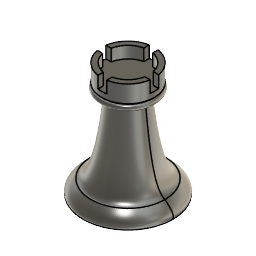
Set sah (Assembly) (Autodesk Fusion 360 archive; units mm, degrees)
design "Tura"
part number: 2026-03-27-15-39-02-789
Autodesk Fusion 360 part; units mm, degrees
sketch "Tura" plane through (0, 0, 0) normal (0, 1, 0) x (1, 0, 0)
  line L0 (0, 0) -> (17, 0)
  line L1 (0, 0) -> (0, -38.5138)
  line L2 (0, -38.5138) -> (0, -35)
  line L3 (0, -38.5138) -> (0, -35)
  line L4 (0, 0) -> (0, -5)
  line L5 (14, -5) -> (0, -5)
  spline S0 degree 5 poles (6.5259, -34) (6.6855, -32.318) (7.0209, -29.0147) (7.5725, -24.2418) (8.412, -18.2671) (9.7194, -11.7648) (11.1016, -7.8229) (12.4226, -5.9311) (13.4497, -5.2188) (14, -5) knots 0 0 0 0 0 0 0.2 0.4 0.6 0.8 1 1 1 1 1 1
  line L6 (12.8092, -5.4735) -> (15.1908, -4.5265)
  spline S1 degree 5 poles (14, -5) (14.3724, -4.7164) (15.065, -4.1591) (15.9469, -3.3525) (16.8041, -2.3367) (17.2264, -1.3701) (17.2496, -0.692) (17.1232, -0.2556) (17.015, -0.0297) (17, 0) knots 0 0 0 0 0 0 0.1 0.2 0.3 0.4 0.415205 0.415205 0.415205 0.415205 0.415205 0.415205
  line L7 (17.1967, -0.3896) -> (16.8033, 0.3896)
  line L8 (0, -37.3622) -> (0, -38.5138)
  line L9 (0, -36) -> (9, -36)
  line L10 (0, -38) -> (0, -36)
  line L11 (8, -40) -> (8, -43)
  line L12 (8, -43) -> (10, -43)
  line L13 (10, -43) -> (10, -36.5)
  line L14 (9.5, -36) -> (9, -36)
  line L15 (0, -36) -> (9.5003, -36)
  line L16 (9.5, -34) -> (0, -34)
  line L17 (0, -34) -> (0, -36)
  arc A0 (9.5005, -34) -> (9.5, -34) centre (9.5, -36.5) ccw
  arc A1 (9.5003, -36) -> (9.5005, -34) centre (9.5003, -35) ccw
  arc A2 (10, -36.5) -> (9.5, -36) centre (9.5, -36.5) ccw
  line L18 (-1.7845, -43) -> (1.4873, -43)
  line L19 (1.4873, -43) -> (1.4873, -38.5138)
  line L20 (1.4873, -38.5138) -> (-1.7845, -38.5138)
  line L21 (-1.7845, -38.5138) -> (-1.7845, -43)
  line L22 (1.4873, -38.5138) -> (8, -38.5138)
  line L23 (8, -38.5138) -> (8, -40)
  point P0 (10, -35)
  dimension "d1" = 17
  dimension "d3" = 10
  dimension "d5" = 3
  dimension "d6" = 2.5
  dimension "d7" = 1
  dimension "d8" = 0.5
  constraint coincident L0.start L1.start
  constraint horizontal L0
  constraint perpendicular L0 L1
  constraint coincident L1 L2.end
  constraint coincident L1 L4.end
  constraint perpendicular L4 L5
  constraint midpoint L5.start L6
  constraint midpoint L0.end L7
  constraint vertical L8
  constraint horizontal L9
  constraint vertical L10
  constraint coincident L1 L9.start
  constraint perpendicular L11 L12
  constraint perpendicular L12 L13
  constraint horizontal L15
  constraint horizontal L16
  constraint vertical L17
  constraint tangent L16 A0
  constraint tangent L15 A1
  constraint tangent A0 A1
  constraint tangent L13 A2
  constraint tangent L14 A2
  constraint coincident S0.start L16
  constraint horizontal L18
  constraint vertical L19
  constraint horizontal L20
  constraint vertical L21
  constraint perpendicular L19 L22
  constraint perpendicular L22 L23
  constraint coincident L20 L1.end
  measures "d1" distance of L0.start L0.end
  measures "d3" distance of L2.end P0
  measures "d5" distance of L11.start L11.end
  measures "d6" radius of A0
  measures "d7" radius of A1
  measures "d8" radius of A2
revolve "Revolve2" add sketch "Tura" angle 360 about axis through (0, 0, 0) along (0, 0, 1) contours L0 L1 L4 L5 S1 | L1 L5 S0 L16 | L1 L2 L3 L9 L15 L16 L17 A0 | L9 L14 L15 A0 A1 | L1 L2 L3 L8 L9 L10 L11 L12 L13 L15 A0 L20 L22 L23 | L9 L13 L14 L15 A0 A2
extrude "Extrude2" cut sketch "Tura" along normal blind 10 contours L18 L19 L20 L21
pattern_circular "C-Pattern1" count 4 over 360 about axis through (0, 0, 0) along (0, 0, 1) of "Extrude2"
named bodies: "Tura"

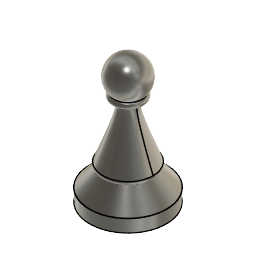
design "Pion"
part number: 2026-03-27-14-13-04-446
Autodesk Fusion 360 part; units mm, degrees
sketch "Pion" plane through (0, 0, 0) normal (0, 1, 0) x (1, 0, 0)
  line L0 (0, 0) -> (12, 0)
  line L1 (12, 0) -> (12, -4) construction
  line L2 (0, 0) -> (0, -40) construction
  line L3 (6, 0) -> (6, -9.5696) construction
  line L4 (0, -30) -> (0, -28) construction
  line L5 (0, -30) -> (4, -30)
  line L6 (0, -28) -> (4, -28)
  arc A0 (4, -30) -> (5, -29) centre (4, -29) ccw
  arc A1 (5, -29) -> (4, -28) centre (4, -29) ccw
  line L7 (12, -4) -> (12, 0)
  line L8 (0, -40) -> (0, 0)
  line L9 (12, -4) -> (0, -4) construction
  line L10 (0, -9.6135) -> (6.9254, -9.6135)
  spline S0 degree 5 poles (7.8558, -10.9801) (7.5549, -11.7439) (6.8618, -13.5183) (5.8277, -16.2235) (4.5513, -19.7052) (3.268, -23.5962) (2.6775, -26.112) (2.6509, -27.3491) (2.8478, -27.8389) (3, -28) knots 0.052342 0.052342 0.052342 0.052342 0.052342 0.052342 0.2 0.4 0.6 0.8 1 1 1 1 1 1
  line L11 (2.6823, -27.6637) -> (3.3177, -28.3363)
  arc A2 (7.8558, -10.9801) -> (6.9254, -9.6135) centre (6.9254, -10.6135) ccw
  spline S1 degree 5 poles (6.9254, -9.6135) (7.1769, -9.3353) (7.6663, -8.794) (8.3596, -8.027) (9.2012, -7.0961) (10.1055, -6.0957) (10.8484, -5.274) (11.4156, -4.6465) (11.7977, -4.2238) (11.9996, -4.0005) (12.0478, -3.9472) (12.0208, -3.977) (12.0038, -3.9958) (12, -4) (12, -4) knots 0 0 0 0 0 0 0.1 0.2 0.3 0.4 0.5 0.6 0.7 0.8 0.9 1 1 1 1 1 1
  line L12 (12.2553, -4.7429) -> (11.7447, -3.257)
  arc A3 (0, -39.9814) -> (4.3789, -29.9254) centre (0, -34) ccw
  dimension "d1" = 12
  dimension "d2" = 4
  dimension "d3" = 40
  dimension "d5" = 2
  dimension "d6" = 1
  dimension "d7" = 1
  constraint coincident L0.start L2.start
  constraint horizontal L0
  constraint perpendicular L0 L1
  constraint perpendicular L0 L2
  constraint midpoint L0 L3.start
  constraint perpendicular L0 L3
  constraint coincident L2 L4.start
  constraint parallel L2 L4
  constraint perpendicular L4 L5
  constraint perpendicular L4 L6
  constraint tangent L5 A0
  constraint tangent L6 A1
  constraint equal A0 A1
  constraint coincident A0.end A1.start
  constraint coincident L1 L7.start
  constraint coincident L2 L9.end
  constraint perpendicular L2 L9
  constraint coincident L8 L10.start
  constraint perpendicular L3 L10
  constraint coincident L6 S0.end
  constraint midpoint S0.end L11
  constraint tangent L10 A2
  constraint tangent S0 A2
  constraint midpoint L1.end L12
  constraint coincident L2 A3.centre
  constraint coincident L2 A3.start
  constraint coincident A0 A3.end
  measures "d1" distance of L0.start L0.end
  measures "d2" distance of L0.end L1.end
  measures "d3" distance of L0.start L2.end
  measures "d5" distance of L4.start L4.end
  measures "d6" radius of A0
  measures "d7" radius of A2
revolve "Revolve1" add sketch "Pion" angle 360 about axis through (0, 0, 40) along (0, 0, -1)
named bodies: "Pion"

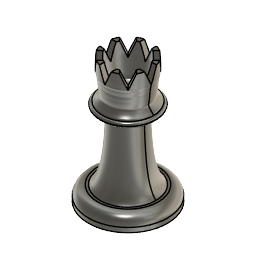
design "Regina"
part number: 2026-03-27-17-57-06-025
Autodesk Fusion 360 part; units mm, degrees
sketch "Regina" plane through (0, 0, 0) normal (0, 1, 0) x (1, 0, 0)
  line L0 (0, 0) -> (17, 0)
  line L1 (0, 0) -> (0, -41)
  line L2 (17, 0) -> (17, -2)
  line L3 (13, -6) -> (0, -6)
  line L4 (0, -41) -> (0, -39.2065) construction
  line L5 (3.0623, -35) -> (0, -35)
  line L6 (0, -35) -> (0, -39.2065)
  arc A0 (13, -6) -> (17, -2) centre (13, -2) ccw
  line L7 (0, -39) -> (0, -41)
  arc A1 (10.0008, -39) -> (10, -39) centre (10, -40) ccw
  line L8 (3.0623, -35) -> (10.9377, -35)
  line L9 (0, -37.1033) -> (10.9434, -37.1033)
  line L10 (11.9419, -36.0482) -> (11.9362, -35.945)
  arc A2 (10.9434, -37.1033) -> (11.9419, -36.0482) centre (10.9434, -36.1033) ccw
  arc A3 (11.9362, -35.945) -> (10.9377, -35) centre (10.9377, -36) ccw
  spline S0 degree 5 poles (0, -41) (0.2083, -40.9398) (0.6157, -40.8267) (1.1995, -40.6787) (1.9231, -40.5249) (2.7363, -40.4049) (3.4584, -40.3568) (4.0905, -40.3792) (4.6342, -40.4699) (5.0924, -40.6251) (5.4693, -40.8395) (5.7707, -41.1057) (6.0047, -41.4142) (6.1808, -41.7532) (6.3098, -42.1104) (6.403, -42.4744) (6.4712, -42.8361) (6.5241, -43.1902) (6.5701, -43.5357) (6.6153, -43.8747) (6.6643, -44.2102) (6.7194, -44.545) (6.7805, -44.8795) (6.8453, -45.2114) (6.9105, -45.5373) (6.9731, -45.8546) (7.0311, -46.1635) (7.085, -46.4688) (7.138, -46.7792) (7.1936, -47.1039) (7.2549, -47.4491) (7.3229, -47.8152) (7.3951, -48.1929) (7.4664, -48.5665) (7.531, -48.9193) (7.5841, -49.2385) (7.6231, -49.5189) (7.6499, -49.7696) (7.6697, -50.0089) (7.6883, -50.2559) (7.711, -50.5249) (7.7399, -50.8159) (7.7746, -51.1193) (7.8131, -51.4217) (7.8528, -51.7111) (7.8909, -51.9831) (7.9257, -52.2421) (7.9554, -52.4973) (7.9791, -52.7592) (7.9959, -53.0363) (8.0054, -53.3331) (8.007, -53.5884) (8.0048, -53.7902) (8.0019, -53.9293) (8, -54) knots 0 0 0 0 0 0 0.02 0.04 0.06 0.08 0.1 0.12 0.14 0.16 0.18 0.2 0.22 0.24 0.26 0.28 0.3 0.32 0.34 0.36 0.38 0.4 0.42 0.44 0.46 0.48 0.5 0.52 0.54 0.56 0.58 0.6 0.62 0.64 0.66 0.68 0.7 0.72 0.74 0.76 0.78 0.8 0.82 0.84 0.86 0.88 0.9 0.92 0.94 0.96 0.98 1 1 1 1 1 1
  line L11 (8, -54) -> (10, -54)
  spline S1 degree 5 poles (10, -54) (10.0003, -53.9643) (10.0009, -53.893) (10.0015, -53.7863) (10.0021, -53.6443) (10.0022, -53.4675) (10.0017, -53.2913) (10.0008, -53.1155) (9.9996, -52.94) (9.9984, -52.7646) (9.9975, -52.5889) (9.9973, -52.4126) (9.9978, -52.2353) (9.9993, -52.057) (10.0013, -51.8776) (10.0035, -51.6974) (10.0048, -51.5172) (10.0047, -51.3382) (10.003, -51.1625) (9.9998, -50.9932) (9.9971, -50.8349) (9.9962, -50.6912) (9.997, -50.5614) (9.999, -50.4427) (10.001, -50.3302) (10.0023, -50.218) (10.0027, -50.0997) (10.0018, -49.9699) (9.9999, -49.825) (9.9968, -49.6648) (9.9924, -49.4929) (9.9865, -49.3152) (9.9792, -49.1386) (9.971, -48.9695) (9.9624, -48.8122) (9.9548, -48.6674) (9.9498, -48.5327) (9.9485, -48.4043) (9.9508, -48.2781) (9.9552, -48.1515) (9.9578, -48.0242) (9.9542, -47.8975) (9.9404, -47.7728) (9.9147, -47.6506) (9.8786, -47.5297) (9.8367, -47.407) (9.7944, -47.2791) (9.7566, -47.1427) (9.7263, -46.9962) (9.7031, -46.8396) (9.685, -46.6745) (9.6688, -46.5033) (9.6514, -46.3293) (9.6302, -46.1561) (9.6043, -45.9872) (9.5742, -45.8253) (9.5412, -45.6726) (9.5073, -45.5295) (9.4745, -45.3949) (9.4447, -45.2651) (9.4194, -45.1349) (9.3997, -44.999) (9.3857, -44.8526) (9.3769, -44.6934) (9.3716, -44.522) (9.3676, -44.341) (9.3626, -44.1544) (9.3546, -43.9664) (9.3422, -43.781) (9.3251, -43.6008) (9.3045, -43.4266) (9.2819, -43.2581) (9.2593, -43.0941) (9.2383, -42.9328) (9.22, -42.7721) (9.2045, -42.6102) (9.1909, -42.4455) (9.1778, -42.2768) (9.1638, -42.1036) (9.1473, -41.9261) (9.1273, -41.7453) (9.1032, -41.5633) (9.0751, -41.3824) (9.0431, -41.2052) (9.0082, -41.0339) (8.9713, -40.8699) (8.934, -40.7138) (8.898, -40.5652) (8.8656, -40.4228) (8.8396, -40.2852) (8.8232, -40.1502) (8.8205, -40.016) (8.8353, -39.881) (8.8703, -39.7444) (8.9259, -39.607) (8.9989, -39.4716) (9.0821, -39.3435) (9.1671, -39.2279) (9.2462, -39.1285) (9.3149, -39.0458) (9.3748, -38.9745) (9.4331, -38.9045) (9.4986, -38.825) (9.5792, -38.7278) (9.6773, -38.6117) (9.7913, -38.4807) (9.9167, -38.342) (10.0475, -38.2039) (10.1775, -38.0737) (10.302, -37.9554) (10.4179, -37.8484) (10.5238, -37.7498) (10.6193, -37.655) (10.7045, -37.5589) (10.7796, -37.4576) (10.8449, -37.3489) (10.8892, -37.2551) (10.918, -37.1808) (10.9352, -37.1294) (10.9434, -37.1033) knots 0 0 0 0 0 0 0.00869565 0.0173913 0.02608696 0.03478261 0.04347826 0.05217391 0.06086957 0.06956522 0.07826087 0.08695652 0.09565217 0.10434783 0.11304348 0.12173913 0.13043478 0.13913043 0.14782609 0.15652174 0.16521739 0.17391304 0.1826087 0.19130435 0.2 0.20869565 0.2173913 0.22608696 0.23478261 0.24347826 0.25217391 0.26086957 0.26956522 0.27826087 0.28695652 0.29565217 0.30434783 0.31304348 0.32173913 0.33043478 0.33913043 0.34782609 0.35652174 0.36521739 0.37391304 0.3826087 0.39130435 0.4 0.40869565 0.4173913 0.42608696 0.43478261 0.44347826 0.45217391 0.46086957 0.46956522 0.47826087 0.48695652 0.49565217 0.50434783 0.51304348 0.52173913 0.53043478 0.53913043 0.54782609 0.55652174 0.56521739 0.57391304 0.5826087 0.59130435 0.6 0.60869565 0.6173913 0.62608696 0.63478261 0.64347826 0.65217391 0.66086957 0.66956522 0.67826087 0.68695652 0.69565217 0.70434783 0.71304348 0.72173913 0.73043478 0.73913043 0.74782609 0.75652174 0.76521739 0.77391304 0.7826087 0.79130435 0.8 0.80869565 0.8173913 0.82608696 0.83478261 0.84347826 0.85217391 0.86086957 0.86956522 0.87826087 0.88695652 0.89565217 0.90434783 0.91304348 0.92173913 0.93043478 0.93913043 0.94782609 0.95652174 0.96521739 0.97391304 0.9826087 0.99130435 1 1 1 1 1 1
  line L12 (10.0315, -52.8303) -> (9.9685, -49.1697)
  line L13 (-1.0096, -55) -> (-3, -55) construction
  line L14 (-3, -55) -> (-1.0096, -55) construction
  line L15 (-3, -55) -> (3, -55)
  line L16 (-3, -55) -> (0, -48)
  line L17 (0, -48) -> (3, -55)
  spline S2 degree 5 poles (7, -35) (7.0241, -33.463) (7.0927, -30.4328) (7.257, -26.0189) (7.6072, -20.4148) (8.3706, -14.1076) (9.4058, -9.9718) (10.541, -7.6389) (11.4828, -6.4802) (12, -6) knots 0 0 0 0 0 0 0.2 0.4 0.6 0.8 1 1 1 1 1 1
  line L18 (10.7838, -7.1292) -> (13.2162, -4.8708)
  point P0 (5.6353, -41)
  point P1 (6.4544, -42.7608)
  point P2 (6.7049, -44.4511)
  point P3 (7, -46)
  point P4 (7.2683, -47.5188)
  point P5 (7.5908, -49.2968)
  point P6 (7.6929, -50.3049)
  point P7 (7.8324, -51.5607)
  point P8 (7.9675, -52.6412)
  point P9 (10, -53)
  point P10 (10, -52)
  point P11 (10, -51)
  point P12 (10, -50.3822)
  point P13 (10, -49.8453)
  point P14 (9.9685, -48.9259)
  point P15 (9.951, -48.2884)
  point P16 (9.9322, -47.743)
  point P17 (9.7687, -47.1812)
  point P18 (9.6508, -46.3325)
  point P19 (9.5, -45.5)
  point P20 (9.3886, -44.8701)
  point P21 (9.3475, -43.8691)
  point P22 (9.2378, -42.9231)
  point P23 (9.1555, -42.0181)
  point P24 (9, -41)
  point P25 (8.8377, -40.2561)
  point P26 (8.9191, -39.6317)
  point P27 (9.2788, -39.0895)
  point P28 (9.5164, -38.8037)
  point P29 (10.1272, -38.125)
  point P30 (10.6702, -37.5956)
  dimension "d1" = 17
  dimension "d4" = 4
  dimension "d7" = 1
  constraint coincident L0.start L1.start
  constraint horizontal L0
  constraint perpendicular L0 L1
  constraint perpendicular L0 L2
  constraint coincident L1 L3.end
  constraint perpendicular L1 L3
  constraint coincident L1 L4.end
  constraint horizontal L5
  constraint vertical L6
  constraint tangent L2 A0
  constraint tangent L3 A0
  constraint vertical L7
  constraint parallel L5 L8
  constraint midpoint L6 L9.start
  constraint perpendicular L1 L9
  constraint tangent L9 A2
  constraint tangent L10 A2
  constraint tangent L8 A3
  constraint tangent L10 A3
  constraint equal A2 A3
  constraint horizontal L11
  constraint midpoint P11 L12
  constraint horizontal L13
  constraint parallel L14 L15
  constraint midpoint L8 S2.start
  constraint coincident L3 S2.end
  constraint midpoint S2.end L18
  measures "d1" distance of L0.start L0.end
  measures "d4" radius of A0
  measures "d7" radius of A2
revolve "Revolve2" add sketch "Regina" angle 360 about axis through (0, 0, 0) along (0, 0, 1) contours L0 L1 L2 L3 A0 | L1 L3 L5 L8 S2 | L1 L5 L6 L8 L9 L10 A2 A3 | L1 L6 L7 L9 S0 L11 S1
extrude "Extrude3" cut sketch "Regina" along normal blind 14 contours L15 L16 L17
pattern_circular "C-Pattern3" count 8 over 360 about axis through (0, 0, 37.1033) along (0, 0, 1) of "Extrude3"
named bodies: "Regina"

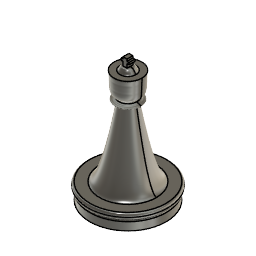
design "Rege"
part number: 2026-03-27-19-00-09-599
Autodesk Fusion 360 part; units mm, degrees
sketch "Rege" plane through (0, 0, 0) normal (0, 1, 0) x (1, 0, 0)
  line L0 (0, 0) -> (19, 0)
  line L1 (0, 0) -> (0, -60)
  line L2 (0, 0) -> (19, 0)
  line L3 (19, 0) -> (19, -4)
  line L4 (18, -5) -> (0, -5)
  line L5 (0, -5) -> (0, 0)
  line L6 (0, -5) -> (19, -5)
  line L7 (18.9974, -7.9995) -> (0, -7.9995)
  line L8 (0, -7.9995) -> (0, -5)
  arc A0 (18.9974, -7.9995) -> (19.8649, -6.502) centre (18.9974, -6.9995) ccw
  arc A1 (19.8649, -6.502) -> (19, -5) centre (19, -6) ccw
  arc A2 (18, -5) -> (19, -4) centre (18, -4) ccw
  line L9 (0, -60) -> (0, -48)
  line L10 (0, -60) -> (0, -40)
  line L11 (0, -37.8406) -> (0, -40)
  line L12 (0, -40) -> (0, -43.0218)
  line L13 (0, -44.611) -> (4.5124, -44.611)
  line L14 (0, -43.0218) -> (0, -44.611)
  spline S0 degree 5 poles (4.3, -42.4) (4.5854, -40.7333) (5.1533, -37.4872) (5.9962, -32.8797) (7.1016, -27.2682) (8.4509, -21.2027) (9.7649, -16.1777) (11.041, -12.29) (12.2781, -9.611) (13.4785, -8.1257) (14.6503, -7.6865) (15.5797, -7.8283) (16.2833, -7.9459) (16.757, -7.9878) (16.995, -7.9995) knots 0 0 0 0 0 0 0.1 0.2 0.3 0.4 0.5 0.6 0.7 0.8 0.9 1 1 1 1 1 1
  line L15 (13.1828, -7.8119) -> (20.8072, -8.1871)
  line L16 (0, -62) -> (1, -62)
  line L17 (1, -62) -> (1, -61)
  line L18 (1, -61) -> (2, -61)
  line L19 (2, -61) -> (2, -60)
  line L20 (2, -60) -> (1, -60)
  line L21 (1, -60) -> (1, -58)
  line L22 (1, -58) -> (0, -58)
  line L23 (0, -60) -> (0, -62)
  spline S1 degree 5 poles (1, -58) (1.0261, -58.002) (1.0784, -58.0057) (1.157, -58.0102) (1.2626, -58.0139) (1.3953, -58.0148) (1.5285, -58.0119) (1.6613, -58.0054) (1.7923, -57.9951) (1.9194, -57.9812) (2.0399, -57.9637) (2.1511, -57.9425) (2.2509, -57.9175) (2.3386, -57.8882) (2.4148, -57.8537) (2.4825, -57.8127) (2.5449, -57.7643) (2.6056, -57.7078) (2.6673, -57.6437) (2.731, -57.5736) (2.7967, -57.4997) (2.8633, -57.4243) (2.9296, -57.3492) (2.9944, -57.2749) (3.0568, -57.2001) (3.1167, -57.1232) (3.174, -57.0419) (3.2294, -56.9548) (3.284, -56.8615) (3.3394, -56.7629) (3.3975, -56.6609) (3.4601, -56.5577) (3.529, -56.4553) (3.6054, -56.3556) (3.6901, -56.2596) (3.7837, -56.1679) (3.8657, -56.0984) (3.9313, -56.0483) (3.9768, -56.016) (4, -56) knots 0 0 0 0 0 0 0.028571 0.057143 0.085714 0.114286 0.142857 0.171429 0.2 0.228571 0.257143 0.285714 0.314286 0.342857 0.371429 0.4 0.428571 0.457143 0.485714 0.514286 0.542857 0.571429 0.6 0.628571 0.657143 0.685714 0.714286 0.742857 0.771429 0.8 0.828571 0.857143 0.885714 0.914286 0.942857 0.971429 1 1 1 1 1 1
  line L24 (4, -56) -> (7, -56)
  spline S2 degree 5 poles (4.5124, -44.611) (4.5363, -44.6464) (4.5836, -44.7159) (4.6528, -44.8164) (4.7418, -44.9431) (4.8473, -45.0892) (4.9477, -45.2239) (5.0436, -45.3482) (5.1363, -45.4642) (5.2275, -45.575) (5.3196, -45.6843) (5.4142, -45.7953) (5.5127, -45.9104) (5.6149, -46.0299) (5.7192, -46.1519) (5.823, -46.2737) (5.9236, -46.3925) (6.0183, -46.5068) (6.1055, -46.6173) (6.1842, -46.7269) (6.2544, -46.8393) (6.3163, -46.9576) (6.3707, -47.0832) (6.4186, -47.2156) (6.461, -47.3527) (6.499, -47.4924) (6.5334, -47.6329) (6.5651, -47.7744) (6.5944, -47.9176) (6.6216, -48.0643) (6.6465, -48.216) (6.6688, -48.3742) (6.6877, -48.5393) (6.7026, -48.7114) (6.7132, -48.8904) (6.7193, -49.0755) (6.722, -49.266) (6.7227, -49.4608) (6.7233, -49.6587) (6.7255, -49.8585) (6.7307, -50.0587) (6.7396, -50.2577) (6.7516, -50.4538) (6.7655, -50.6453) (6.7796, -50.831) (6.7923, -51.0103) (6.8026, -51.1836) (6.8102, -51.3526) (6.8158, -51.5199) (6.8207, -51.6886) (6.8259, -51.8614) (6.8323, -52.0401) (6.8399, -52.2248) (6.8478, -52.4137) (6.8548, -52.6045) (6.8598, -52.7945) (6.8622, -52.9814) (6.8623, -53.1645) (6.8615, -53.3447) (6.862, -53.5237) (6.866, -53.704) (6.8752, -53.8879) (6.8906, -54.0768) (6.9114, -54.2708) (6.9362, -54.469) (6.9623, -54.6696) (6.9871, -54.8706) (7.008, -55.0699) (7.0229, -55.266) (7.0304, -55.4576) (7.0296, -55.6442) (7.0222, -55.7893) (7.0126, -55.8956) (7.0045, -55.9654) (7, -56) knots 0 0 0 0 0 0 0.01428571 0.02857143 0.04285714 0.05714286 0.07142857 0.08571429 0.1 0.11428571 0.12857143 0.14285714 0.15714286 0.17142857 0.18571429 0.2 0.21428571 0.22857143 0.24285714 0.25714286 0.27142857 0.28571429 0.3 0.31428571 0.32857143 0.34285714 0.35714286 0.37142857 0.38571429 0.4 0.41428571 0.42857143 0.44285714 0.45714286 0.47142857 0.48571429 0.5 0.51428571 0.52857143 0.54285714 0.55714286 0.57142857 0.58571429 0.6 0.61428571 0.62857143 0.64285714 0.65714286 0.67142857 0.68571429 0.7 0.71428571 0.72857143 0.74285714 0.75714286 0.77142857 0.78571429 0.8 0.81428571 0.82857143 0.84285714 0.85714286 0.87142857 0.88571429 0.9 0.91428571 0.92857143 0.94285714 0.95714286 0.97142857 0.98571429 1 1 1 1 1 1
  line L25 (11, -41.5218) -> (11, -41.5)
  line L26 (0, -42.4) -> (4.7, -42.4)
  line L27 (0, -44.611) -> (4.5124, -44.611)
  spline S3 degree 5 poles (4.5124, -44.611) (4.5154, -44.5998) (4.5227, -44.5779) (4.5373, -44.5462) (4.5641, -44.5064) (4.6099, -44.4604) (4.6672, -44.4181) (4.7346, -44.3788) (4.8099, -44.3414) (4.8897, -44.3046) (4.971, -44.2668) (5.0508, -44.2273) (5.1275, -44.1854) (5.2013, -44.1421) (5.274, -44.0992) (5.3486, -44.0588) (5.428, -44.0231) (5.514, -43.9937) (5.6068, -43.9707) (5.7039, -43.9528) (5.8016, -43.9376) (5.8956, -43.9226) (5.9825, -43.9055) (6.0599, -43.8852) (6.1285, -43.8623) (6.1907, -43.8388) (6.2497, -43.8166) (6.3077, -43.7971) (6.3652, -43.7795) (6.4194, -43.7609) (6.4664, -43.7371) (6.502, -43.7046) (6.5232, -43.6622) (6.5297, -43.6119) (6.523, -43.5581) (6.5052, -43.5053) (6.4782, -43.4569) (6.4424, -43.4129) (6.397, -43.3711) (6.3413, -43.3284) (6.2746, -43.2819) (6.1975, -43.2306) (6.1117, -43.1754) (6.0196, -43.1187) (5.924, -43.0634) (5.8277, -43.0123) (5.7327, -42.9673) (5.64, -42.9285) (5.5496, -42.8945) (5.4611, -42.8628) (5.3731, -42.8306) (5.2847, -42.7948) (5.1946, -42.7526) (5.1021, -42.7024) (5.0067, -42.6428) (4.9081, -42.5731) (4.8266, -42.5091) (4.7639, -42.4564) (4.7214, -42.4191) (4.7, -42.4) knots 0 0 0 0 0 0 0.018182 0.036364 0.054545 0.072727 0.090909 0.109091 0.127273 0.145455 0.163636 0.181818 0.2 0.218182 0.236364 0.254545 0.272727 0.290909 0.309091 0.327273 0.345455 0.363636 0.381818 0.4 0.418182 0.436364 0.454545 0.472727 0.490909 0.509091 0.527273 0.545455 0.563636 0.581818 0.6 0.618182 0.636364 0.654545 0.672727 0.690909 0.709091 0.727273 0.745455 0.763636 0.781818 0.8 0.818182 0.836364 0.854545 0.872727 0.890909 0.909091 0.927273 0.945455 0.963636 0.981818 1 1 1 1 1 1
  line L28 (0, -62) -> (-1, -62)
  line L29 (-1, -62) -> (-1, -61)
  line L30 (-1, -61) -> (-2, -61)
  line L31 (-2, -61) -> (-2, -60)
  line L32 (-2, -60) -> (-1, -60)
  line L33 (-1, -60) -> (-1, -58)
  line L34 (-1, -58) -> (0, -58)
  point P0 (14.0855, -7.9995)
  point P1 (1.7236, -58)
  point P2 (2.3, -57.9)
  point P3 (2.6058, -57.706)
  point P4 (2.91, -57.3713)
  point P5 (3.2, -57)
  point P6 (3.5, -56.5)
  point P7 (5.0617, -45.3702)
  point P8 (5.4826, -45.8753)
  point P9 (5.9597, -46.4365)
  point P10 (6.2959, -46.9218)
  point P11 (6.5, -47.5)
  point P12 (6.6352, -48.1496)
  point P13 (6.716, -48.9897)
  point P14 (6.7321, -50.0721)
  point P15 (6.7967, -51.0899)
  point P16 (6.8291, -51.9461)
  point P17 (6.8614, -52.9478)
  point P18 (6.8775, -53.9009)
  point P19 (7, -55)
  point P20 (4.7, -44.4)
  point P21 (5.1, -44.2)
  point P22 (5.5, -44)
  point P23 (6, -43.9)
  point P24 (6.3, -43.8)
  point P25 (6.5, -43.7)
  point P26 (6.5, -43.5)
  point P27 (6.3, -43.3)
  point P28 (5.8, -43)
  point P29 (5.3, -42.8)
  dimension "d1" = 19
  dimension "d2" = 1
  dimension "d3" = 20
  dimension "d5" = 2
  constraint coincident L0.start L1.start
  constraint horizontal L0
  constraint perpendicular L0 L1
  constraint horizontal L2
  constraint vertical L3
  constraint horizontal L4
  constraint vertical L5
  constraint horizontal L6
  constraint horizontal L7
  constraint vertical L8
  constraint tangent L7 A0
  constraint tangent L6 A1
  constraint equal A0 A1
  constraint coincident A0.end A1.start
  constraint tangent L3 A2
  constraint tangent L4 A2
  constraint equal A0 A2
  constraint coincident L1 L9.end
  constraint parallel L1 L10
  constraint vertical L11
  constraint vertical L12
  constraint coincident L1 L12.end
  constraint horizontal L13
  constraint vertical L14
  constraint coincident L1 L13.start
  constraint coincident L7 S0.end
  constraint midpoint S0.end L15
  constraint perpendicular L10 L16
  constraint perpendicular L16 L17
  constraint perpendicular L17 L18
  constraint perpendicular L18 L19
  constraint perpendicular L17 L20
  constraint perpendicular L20 L21
  constraint coincident L10 L22.end
  constraint perpendicular L16 L23
  constraint perpendicular L9 L24
  constraint coincident L7 P0
  constraint coincident L1 L26.start
  constraint perpendicular L12 L26
  constraint perpendicular L1 L27
  constraint coincident S0.start L26
  constraint perpendicular L23 L28
  constraint perpendicular L28 L29
  constraint perpendicular L29 L30
  constraint perpendicular L30 L31
  constraint perpendicular L31 L32
  constraint perpendicular L32 L33
  constraint perpendicular L10 L34
  measures "d1" distance of L0.start L0.end
  measures "d2" radius of A0
  measures "d3" distance of L1.end L10.end
  measures "d5" distance of L20.end L21.end
revolve "Revolve1" add sketch "Rege" angle 360 about axis through (0, 0, 0) along (0, 0, 1) contours L0 L1 L2 L3 L4 L5 L6 A2 | L1 L4 L6 L7 L8 A0 A1 S0 L15 | L1 L7 L10 L11 L12 S0 L26 | L1 L10 L12 L13 L14 L26 L27 S3 | L1 L9 L10 L13 L22 S1 L24 S2 L27 picked at (12.3333, -1.6667) picked at (10.6952, -5.9998) picked at (2.9652, -21.8232) picked at (2.9417, -43.3323) picked at (3.5718, -50.9916)
extrude "Extrude1" add sketch "Rege" along normal blind 1.5 and the other way blind 1.5 contours L1 L9 L10 L16 L17 L18 L19 L20 L21 L22 L23 | L1 L9 L10 L23 L28 L29 L30 L31 L32 L33 L34 picked at (0.3333, -61) picked at (-0.3333, -61)
named bodies: "Rege"

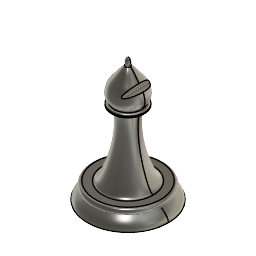
design "Nebun"
part number: 2026-03-27-16-39-54-698
Autodesk Fusion 360 part; units mm, degrees
sketch "Nebun" plane through (0, 0, 0) normal (0, 1, 0) x (1, 0, 0)
  line L0 (0, 0) -> (0, -46.4544)
  line L1 (0, -46.4544) -> (0, -45.1268) construction
  line L2 (0, -35) -> (0, -45.1268)
  arc A0 (0, -46.4544) -> (1, -46) centre (0, -45.1268) ccw
  line L3 (0, -32.0025) -> (3.4069, -32.0025)
  line L4 (3.4069, -32.0025) -> (5.4675, -32.0025)
  line L5 (9.9478, -6.4764) -> (0, -6.4764)
  line L6 (0, -49) -> (0, -46.4544)
  spline S0 degree 5 poles (0, -46.4544) (0.0754, -46.4311) (0.2198, -46.3948) (0.4172, -46.3713) (0.641, -46.4028) (0.8509, -46.5512) (0.9847, -46.8088) (1.036, -47.1672) (1.0017, -47.5979) (0.8824, -48.0528) (0.6792, -48.4775) (0.4497, -48.7506) (0.2397, -48.8993) (0.0827, -48.971) (0, -49) knots 0 0 0 0 0 0 0.1 0.2 0.3 0.4 0.5 0.6 0.7 0.8 0.9 1 1 1 1 1 1
  line L7 (0.2729, -48.9043) -> (-0.2729, -49.0957)
  line L8 (0, 0) -> (16, 0)
  line L9 (0, -6.4764) -> (12.9366, -6.4764)
  line L10 (12.9366, -4.0764) -> (0, -4.0764)
  line L11 (0, -4.0764) -> (0, -6.4764)
  arc A1 (12.9366, -6.4764) -> (14.1366, -5.2855) centre (12.9366, -5.2764) ccw
  arc A2 (14.1366, -5.2855) -> (12.9366, -4.0764) centre (12.9366, -5.2764) ccw
  spline S1 degree 5 poles (12.9366, -4.0764) (13.1271, -3.9343) (13.5002, -3.6476) (14.0361, -3.2102) (14.7, -2.6114) (15.4041, -1.8243) (15.8034, -1.1441) (15.9642, -0.5913) (16, -0.2008) (16, 0) knots 0 0 0 0 0 0 0.2 0.4 0.6 0.8 1 1 1 1 1 1
  line L12 (16, -0.463) -> (16, 0.463)
  line L13 (0, -33.5564) -> (5.4675, -33.5564)
  spline S2 degree 5 poles (1, -46) (1.0428, -45.9606) (1.127, -45.8825) (1.2496, -45.7674) (1.4055, -45.6178) (1.5877, -45.4373) (1.7578, -45.2628) (1.917, -45.0931) (2.0669, -44.9266) (2.2103, -44.7605) (2.3506, -44.5914) (2.4916, -44.4159) (2.6365, -44.2312) (2.7873, -44.0357) (2.9446, -43.8302) (3.107, -43.6175) (3.2717, -43.4017) (3.4359, -43.1875) (3.5967, -42.9791) (3.7521, -42.7796) (3.9018, -42.5897) (4.047, -42.4082) (4.1899, -42.2323) (4.3327, -42.0587) (4.4778, -41.884) (4.6264, -41.705) (4.7787, -41.5199) (4.9342, -41.3276) (5.0913, -41.128) (5.2481, -40.9217) (5.402, -40.7106) (5.5503, -40.4973) (5.6899, -40.285) (5.8185, -40.0766) (5.9341, -39.8743) (6.0357, -39.6789) (6.1236, -39.4894) (6.1993, -39.3029) (6.2652, -39.1158) (6.3237, -38.9245) (6.3773, -38.726) (6.4282, -38.519) (6.4776, -38.3035) (6.5263, -38.081) (6.5739, -37.8538) (6.619, -37.6253) (6.6591, -37.3992) (6.691, -37.1796) (6.712, -36.9697) (6.7203, -36.7711) (6.7158, -36.5835) (6.701, -36.4038) (6.6795, -36.2273) (6.6541, -36.05) (6.6259, -35.8693) (6.5924, -35.686) (6.5483, -35.5037) (6.4876, -35.3265) (6.4054, -35.1579) (6.3, -34.9985) (6.1733, -34.8459) (6.0294, -34.6971) (5.8729, -34.5499) (5.7084, -34.4052) (5.5382, -34.2692) (5.363, -34.1508) (5.1825, -34.0577) (4.9957, -33.9928) (4.8019, -33.95) (4.6011, -33.911) (4.3938, -33.8513) (4.2232, -33.7669) (4.0929, -33.6741) (4.0051, -33.598) (3.9609, -33.5564) knots 0 0 0 0 0 0 0.01428571 0.02857143 0.04285714 0.05714286 0.07142857 0.08571429 0.1 0.11428571 0.12857143 0.14285714 0.15714286 0.17142857 0.18571429 0.2 0.21428571 0.22857143 0.24285714 0.25714286 0.27142857 0.28571429 0.3 0.31428571 0.32857143 0.34285714 0.35714286 0.37142857 0.38571429 0.4 0.41428571 0.42857143 0.44285714 0.45714286 0.47142857 0.48571429 0.5 0.51428571 0.52857143 0.54285714 0.55714286 0.57142857 0.58571429 0.6 0.61428571 0.62857143 0.64285714 0.65714286 0.67142857 0.68571429 0.7 0.71428571 0.72857143 0.74285714 0.75714286 0.77142857 0.78571429 0.8 0.81428571 0.82857143 0.84285714 0.85714286 0.87142857 0.88571429 0.9 0.91428571 0.92857143 0.94285714 0.95714286 0.97142857 0.98571429 1 1 1 1 1 1
  line L14 (5.5565, -35.059) -> (2.3653, -32.0538)
  line L15 (6.4675, -32.5564) -> (6.4675, -33.0025)
  arc A3 (5.4675, -33.5564) -> (6.4675, -32.5564) centre (5.4675, -32.5564) ccw
  arc A4 (6.4675, -33.0025) -> (5.4675, -32.0025) centre (5.4675, -33.0025) ccw
  spline S3 degree 5 poles (4.4372, -32.0025) (4.3926, -31.7636) (4.3089, -31.2754) (4.1994, -30.5122) (4.0855, -29.4321) (3.9996, -27.9741) (3.9765, -26.4008) (4.0266, -24.702) (4.1657, -22.8634) (4.4123, -20.8737) (4.7831, -18.7344) (5.2885, -16.4691) (5.9279, -14.1341) (6.6841, -11.8299) (7.5173, -9.7149) (8.3754, -7.9746) (9.04, -7.0247) (9.5079, -6.6229) (9.8038, -6.501) (9.9478, -6.4764) knots 0 0 0 0 0 0 0.066667 0.133333 0.2 0.266667 0.333333 0.4 0.466667 0.533333 0.6 0.666667 0.733333 0.8 0.866667 0.933333 1 1 1 1 1 1
  line L16 (8.9423, -6.6477) -> (10.9532, -6.3052)
  spline S4 degree 5 poles (4.4165, -41.9579) (4.2811, -41.7738) (4.0247, -41.4179) (3.6836, -40.9207) (3.317, -40.3323) (3.0158, -39.7297) (2.8861, -39.2721) (2.9422, -38.9716) (3.1927, -38.8355) (3.6309, -38.8581) (4.2431, -39.0278) (4.8608, -39.2718) (5.3915, -39.5118) (5.7748, -39.6967) (5.9738, -39.7954) knots 0 0 0 0 0 0 0.1 0.2 0.3 0.4 0.5 0.6 0.7 0.8 0.9 1 1 1 1 1 1
  point P0 (9.9942, -32.0025)
  point P1 (9.994, -33.0025)
  point P2 (2, -45)
  point P3 (2.7357, -44.1024)
  point P4 (3.6547, -42.9048)
  point P5 (4.4165, -41.9579)
  point P6 (5.2422, -40.9275)
  point P7 (5.9738, -39.7954)
  point P8 (6.3277, -38.9044)
  point P9 (6.5754, -37.8427)
  point P10 (6.717, -36.7809)
  point P11 (6.6462, -36.0022)
  point P12 (6.4339, -35.2236)
  point P13 (5.8322, -34.5157)
  point P14 (5, -34)
  point P15 (4, -26)
  point P16 (6, -14)
  point P17 (1, -47)
  point P18 (3, -39)
  dimension "d8" = 1
  dimension "d11" = 16
  dimension "d12" = 1.2
  dimension "d14" = 1
  dimension "d21" = 49
  constraint coincident L0.start L8.start
  constraint parallel L0 L1
  constraint vertical L2
  constraint coincident L1.end L2.end
  constraint coincident L0 L3.start
  constraint perpendicular L0 L3
  constraint parallel L3 L4
  constraint coincident P0 L4
  constraint coincident L0 L5.end
  constraint perpendicular L0 L5
  constraint coincident L4 S3.start
  constraint coincident L6.start S0.end
  constraint parallel L1 L6
  constraint midpoint L6.start L7
  constraint perpendicular L0 L8
  constraint horizontal L9
  constraint horizontal L10
  constraint vertical L11
  constraint tangent L9 A1
  constraint tangent L10 A2
  constraint equal A1 A2
  constraint midpoint L8.end L12
  constraint coincident L0 L13.start
  constraint perpendicular L0 L13
  constraint coincident L13 S2.end
  constraint midpoint S2.end L14
  constraint perpendicular L4 L15
  constraint tangent L13 A3
  constraint tangent L15 A3
  constraint tangent L4 A4
  constraint tangent L15 A4
  constraint equal A3 A4
  constraint midpoint L5.start L16
  constraint coincident P5 S4.start
  constraint coincident P7 S4.end
  measures "d8" distance of P0 P1
  measures "d11" distance of L0.start L8.end
  measures "d12" radius of A1
  measures "d14" radius of A3
  measures "d21" distance of L0.start L6.start
revolve "Revolve2" add sketch "Nebun" angle 360 about axis through (0, 0, 0) along (0, 0, 1)
extrude "Extrude1" cut sketch "Nebun" along normal blind 6 contours S2 S4
extrude "Extrude2" cut sketch "Nebun" against normal blind 6 contours S2 S4
named bodies: "Nebun"
